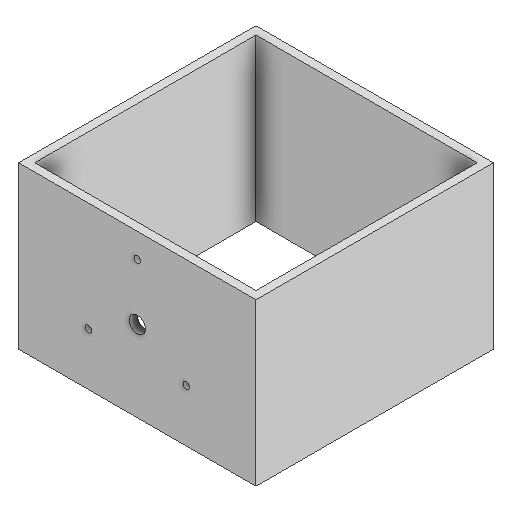
# Autodesk Inventor part: Seccion_tunel
Saved by Autodesk Inventor 2025.2 (Build 292293000, 293)
## iProperties
Created: 2025-05-05
Part Number: Seccion_tunel
Material: Generic
Document SubType Name: Modeling
Designer: nicoa
Density: 1 g/cm^3
Appearance: Default
Author: nicoa
Autodesk Inventor part; units mm, degrees
ref_plane "YZ Plane" through (0, 0, 0) normal (1, 0, 0) x (0, 1, 0)
ref_plane "XZ Plane" through (0, 0, 0) normal (0, 1, 0) x (-1, 0, 0)
ref_plane "XY Plane" through (0, 0, 0) normal (0, 0, 1) x (1, 0, 0)
sketch "Sketch1" plane through (0, 0, 0) normal (0, 1, 0) x (-1, 0, 0)
  line L0 (-68.5, -68.5) -> (68.5, -68.5)
  line L1 (68.5, -68.5) -> (68.5, 68.5)
  line L2 (68.5, 68.5) -> (-68.5, 68.5)
  line L3 (-68.5, 68.5) -> (-68.5, -68.5)
  line L4 (-68.5, -68.5) -> (68.5, 68.5) construction
  line L5 (68.5, -68.5) -> (-68.5, 68.5) construction
  line L6 (-73.5, 73.5) -> (73.5, 73.5)
  line L7 (73.5, 73.5) -> (73.5, -73.5)
  line L8 (73.5, -73.5) -> (-73.5, -73.5)
  line L9 (-73.5, -73.5) -> (-73.5, 73.5)
  point P0 (0, 0)
  dimension "d0" = 137
  dimension "d1" = 137
  dimension "d2" = 5
  constraints: 20 end point, 4 parallel, 2 midpoint, 2 perpendicular, 1 horizontal, 3 other
  measures "d0" distance of L0.end L1.end
  measures "d1" distance of L1.end L2.end
  measures "d2" distance between parallel lines of L2 L6
extrude "Extrusion1" add sketch "Sketch1" along normal blind 100
sketch "Sketch2" plane through (-73.5, 0, 73.5) normal (0, 0, 1) x (1, 0, 0)
  line L0 (0, 0) -> (147, 0) projected
  line L1 (147, 0) -> (147, 100) projected
  line L2 (0, 100) -> (147, 100) projected
  line L3 (0, 0) -> (0, 100) projected
  circle A0 centre (73.5, 50) radius 35
  circle A1 centre (73.5, 85) radius 2
  circle A2 centre (43.1891, 32.5) radius 2
  circle A3 centre (103.8109, 32.5) radius 2
  circle A4 centre (73.5, 50) radius 5
  point P0 (73.5, 0)
  dimension "d5" = 70
  dimension "d6" = 4
  dimension "d9" = 360
  dimension "d13" = 10
  constraints: 4 centre point, 1 coincident, 1 vertical alignment, 9 other
  measures "d6" diameter of A1
  measures "d13" diameter of A4
extrude "Extrusion2" cut sketch "Sketch2" against normal blind 5 contours A1 A0 | A0 A1 | A3 A0 | A0 A3 | A2 A0 | A0 A2 | A4
body "Solid1"
